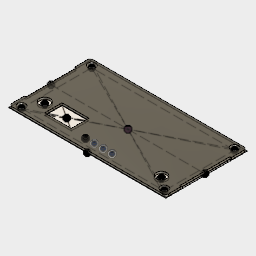
HL2_End_Caps (Autodesk Fusion 360 design; units mm, degrees)
Autodesk Fusion 360 part; units mm, degrees
sketch "Sketch1" plane through (0, 0, 0) normal (0, 0, 1) x (1, 0, 0) in component "Front Cover"
  line L0 (53, 27.5) -> (-53, 27.5)
  line L1 (-53, 27.5) -> (-53, -27.5)
  line L2 (-53, -27.5) -> (53, -27.5)
  line L3 (53, -27.5) -> (53, 27.5)
  line L4 (53, 27.5) -> (-53, -27.5) construction
  line L5 (-53, 27.5) -> (53, -27.5) construction
  line L6 (48.25, 23.75) -> (-48.25, 23.75) construction
  line L7 (-48.25, 23.75) -> (-48.25, -23.75) construction
  line L8 (-48.25, -23.75) -> (48.25, -23.75) construction
  line L9 (48.25, -23.75) -> (48.25, 23.75) construction
  line L10 (48.25, 23.75) -> (-48.25, -23.75) construction
  line L11 (-48.25, 23.75) -> (48.25, -23.75) construction
  circle A0 centre (-48.25, 23.75) radius 1.6
  circle A1 centre (48.25, 23.75) radius 1.6
  circle A2 centre (48.25, -23.75) radius 1.6
  circle A3 centre (-48.25, -23.75) radius 1.6
  line L12 (-53, 0) -> (53, 0) construction
  line L13 (-52, 17) -> (-52, -17)
  line L14 (-52, 17) -> (-53, 17)
  line L15 (-52, -17) -> (-53, -17)
  line L16 (52, 17) -> (52, -17)
  line L17 (52, 17) -> (53, 17)
  line L18 (52, -17) -> (53, -17)
  circle A4 centre (-42.9, -13.35) radius 3.625
  circle A5 centre (39.85, -17.25) radius 3.5
  circle A6 centre (-9, -19.75) radius 1
  circle A7 centre (-3, -19.75) radius 1
  circle A8 centre (3, -19.75) radius 1
  circle A9 centre (9, -19.75) radius 1
  line L19 (-18.25, -20.025) -> (-36.25, -20.025)
  line L20 (-36.25, -20.025) -> (-36.25, -8.275)
  line L21 (-36.25, -8.275) -> (-18.25, -8.275)
  line L22 (-18.25, -8.275) -> (-18.25, -20.025)
  line L23 (-18.25, -20.025) -> (-36.25, -8.275) construction
  line L24 (-36.25, -20.025) -> (-18.25, -8.275) construction
  point P0 (0, -27.5)
  point P1 (-52, 0)
  point P2 (52, 0)
  point P3 (-42.9, -13.35)
  point P4 (39.85, -17.25)
  point P5 (-9, -19.75)
  point P6 (-3, -19.75)
  point P7 (3, -19.75)
  point P8 (9, -19.75)
  point P9 (-27.25, -14.15)
  dimension "d1" = 106
  dimension "d2" = 55
  dimension "d5" = 96.5
  dimension "d6" = 47.5
  dimension "d7" = 3.2
  dimension "d10" = 34
  dimension "d11" = 1
  dimension "d12" = 34
  dimension "d13" = 1
  dimension "d16" = 14.15
  dimension "d17" = 10.1
  dimension "d18" = 7.25
  dimension "d25" = 10.25
  dimension "d26" = 13.15
  dimension "d27" = 7
  dimension "d33" = 7.75
  dimension "d34" = 44
  dimension "d35" = 6
  dimension "d36" = 6
  dimension "d37" = 12
  dimension "d38" = 6
  dimension "d39" = 2
  dimension "d49" = 18
  dimension "d50" = 11.75
  dimension "d51" = 13.35
  dimension "d52" = 25.75
  measures "d1" distance of L1.end L2.end
  measures "d2" distance of L0.end L1.end
  measures "d5" distance of L7.end L8.end
  measures "d6" distance of L6.end L7.end
  measures "d7" diameter of A0
  measures "d10" distance of L13.start L13.end
  measures "d11" distance of L1 L13
  measures "d12" distance of L16.start L16.end
  measures "d13" distance of L3 L16
  measures "d16" distance of L2 P3
  measures "d17" distance of L1 P3
  measures "d18" diameter of A4
  measures "d25" distance of L2 P4
  measures "d26" distance of L3 P4
  measures "d27" diameter of A5
  measures "d33" distance of L2 P5
  measures "d34" distance of L1 P5
  measures "d35" distance of P5 P6
  measures "d36" distance of P6 P7
  measures "d37" distance of P5 P7
  measures "d38" distance of P7 P8
  measures "d39" diameter of A6
  measures "d49" distance of L20.end L21.end
  measures "d50" distance of L19.end L20.end
  measures "d51" distance of L2 P9
  measures "d52" distance of L1 P9
extrude "Extrude5" add sketch "Sketch1" along normal blind 1.5 contours L0 L1 L2 L3 L13 L14 L15 L16 L17 L18 makes body 1 in component "Front Cover"
fillet "Fillet2" radius 2 4 edges at (-53, -27.5, 0.75) (-53, 27.5, 0.75) (53, 27.5, 0.75) (53, -27.5, 0.75) on bodies 1 in component "Front Cover"
chamfer "Chamfer3" distance 1 angle 45 4 edges at (-49.7417, -23.1714, 1.5) (-49.7417, 24.3286, 1.5) (46.7583, 24.3286, 1.5) (46.7583, -23.1714, 1.5) on bodies 1 in component "Front Cover"
sketch "Sketch1 (2)" plane through (0, 0, 0) normal (0, 0, 1) x (1, 0, 0) in component "Rear Cover"
  line L0 (53, 27.5) -> (-53, 27.5)
  line L1 (-53, 27.5) -> (-53, -27.5)
  line L2 (-53, -27.5) -> (53, -27.5)
  line L3 (53, -27.5) -> (53, 27.5)
  line L4 (53, 27.5) -> (-53, -27.5) construction
  line L5 (-53, 27.5) -> (53, -27.5) construction
  line L6 (48.25, 23.75) -> (-48.25, 23.75) construction
  line L7 (-48.25, 23.75) -> (-48.25, -23.75) construction
  line L8 (-48.25, -23.75) -> (48.25, -23.75) construction
  line L9 (48.25, -23.75) -> (48.25, 23.75) construction
  line L10 (48.25, 23.75) -> (-48.25, -23.75) construction
  line L11 (-48.25, 23.75) -> (48.25, -23.75) construction
  circle A0 centre (-48.25, 23.75) radius 1.6
  circle A1 centre (48.25, 23.75) radius 1.6
  circle A2 centre (48.25, -23.75) radius 1.6
  circle A3 centre (-48.25, -23.75) radius 1.6
  line L12 (-53, 0) -> (53, 0) construction
  line L13 (-52, 17) -> (-52, -17)
  line L14 (-52, 17) -> (-53, 17)
  line L15 (-52, -17) -> (-53, -17)
  line L16 (52, 17) -> (52, -17)
  line L17 (52, 17) -> (53, 17)
  line L18 (52, -17) -> (53, -17)
  circle A4 centre (-38, -13.5) radius 4.5
  circle A5 centre (-18, -19.5) radius 3.25
  circle A6 centre (14, -19.5) radius 3.25
  point P0 (0, -27.5)
  point P1 (-52, 0)
  point P2 (52, 0)
  dimension "d1_1" = 106
  dimension "d2_1" = 55
  dimension "d5_1" = 96.5
  dimension "d6_1" = 47.5
  dimension "d7_1" = 3.2
  dimension "d10_1" = 34
  dimension "d11_1" = 1
  dimension "d12_1" = 34
  dimension "d13_1" = 1
  dimension "d53" = 15
  dimension "d54" = 14
  dimension "d55" = 9
  dimension "d56" = 6.5
  dimension "d57" = 35
  dimension "d58" = 8
  dimension "d59" = 67
  measures "d1_1" distance of L1.end L2.end
  measures "d2_1" distance of L0.end L1.end
  measures "d5_1" distance of L7.end L8.end
  measures "d6_1" distance of L6.end L7.end
  measures "d7_1" diameter of A0
  measures "d10_1" distance of L13.start L13.end
  measures "d11_1" distance of L1 L13
  measures "d12_1" distance of L16.start L16.end
  measures "d13_1" distance of L3 L16
  measures "d53" distance of L1 A4.centre
  measures "d54" distance of L2 A4.centre
  measures "d55" diameter of A4
  measures "d56" diameter of A5
  measures "d57" distance of L1 A5.centre
  measures "d58" distance of L2 A5.centre
  measures "d59" distance of L1 A6.centre
extrude "Extrude5'" add sketch "Sketch1 (2)" along normal blind 1.5 separate body contours L0 L1 L2 L3 L13 L14 L15 L16 L17 L18 makes body 2 in component "Rear Cover"
fillet "Fillet2'" radius 2 4 edges at (-53, -27.5, 0.75) (-53, 27.5, 0.75) (53, 27.5, 0.75) (53, -27.5, 0.75) on bodies 2 in component "Rear Cover"
chamfer "Chamfer3'" distance 1 angle 45 4 edges at (-49.7417, -23.1714, 1.5) (-49.7417, 24.3286, 1.5) (46.7583, 24.3286, 1.5) (46.7583, -23.1714, 1.5) on bodies 2 in component "Rear Cover"
component "Front Cover" placed x (1, 0, 0) y (0, 1, 0) z (0, 0, 1) at (0, 0, 0)
component "Rear Cover" placed x (1, 0, 0) y (0, 1, 0) z (0, 0, 1) at (0, 0, 0)
